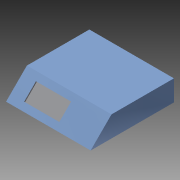
# Autodesk Inventor part: hotbody
Saved by Autodesk Inventor 2014 (Build 180170000, 170)
## iProperties
Created: 2014-07-14
Part Number: hotbody
Material: Generic
Document SubType Name: Modeling
Designer: Nabeel
Density: 1 g/cm^3
Appearance: Default
Author: Nabeel
Autodesk Inventor part; units mm, degrees
ref_plane "YZ Plane" through (0, 0, 0) normal (1, 0, 0) x (0, 1, 0)
ref_plane "XZ Plane" through (0, 0, 0) normal (0, 1, 0) x (-1, 0, 0)
ref_plane "XY Plane" through (0, 0, 0) normal (0, 0, 1) x (1, 0, 0)
sketch "Sketch1" plane through (0, 0, 0) normal (0, 0, 1) x (1, 0, 0)
  line L0 (-40.6, 0) -> (243.6, 0) projected
  line L1 (0, -40) -> (0, 240) projected
  line L2 (0, 0) -> (203, 0)
  line L3 (203, 0) -> (203, 200)
  line L4 (203, 200) -> (0, 200)
  line L5 (0, 200) -> (0, 0)
  dimension "d0" = 203
  dimension "d1" = 200
  constraints: 8 end point, 2 parallel, 1 horizontal, 1 perpendicular
  measures "d0" distance between parallel lines of L3 L5
  measures "d1" distance between parallel lines of L4 L2
extrude "Extrusion1" add sketch "Sketch1" along normal blind 50
chamfer "Chamfer1" distance 50 angle 45 1 edges at (101.5, 0, 50)
sketch "Sketch4" plane through (0, 50, 50) normal (0, -0.7071, 0.7071) x (1, 0, 0)
  line L0 (32.6771, -55.3553) -> (116.9718, -55.3553)
  line L1 (116.9718, -55.3553) -> (116.9718, -15.3553)
  line L2 (116.9718, -15.3553) -> (32.6771, -15.3553)
  line L3 (32.6771, -15.3553) -> (32.6771, -55.3553)
  constraints: 8 end point, 2 parallel, 1 horizontal, 1 perpendicular
extrude "Extrusion4" cut sketch "Sketch4" against normal blind 3
body "Solid1"
